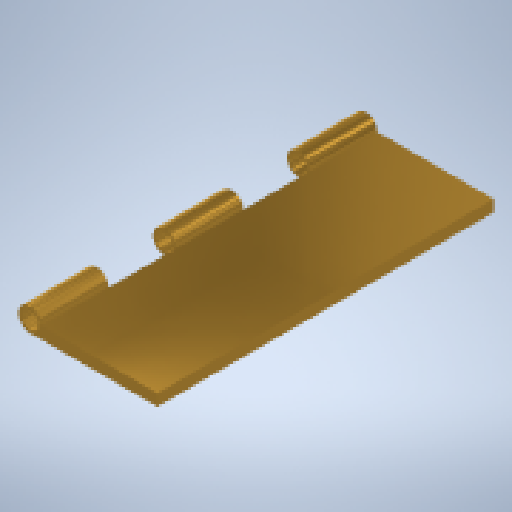
# Autodesk Inventor part: SchnierTeilA
Saved by Autodesk Inventor 2024 (Build 280153000, 153)
## iProperties
Created: 2023-11-30
Part Number: SchnierTeilA
Material: Generic
Document SubType Name: Modeling
Designer: Daniel Nussbaum
Density: 1 g/cm^3
Appearance: Default
Author: Daniel Nussbaum
Autodesk Inventor part; units mm, degrees
ref_plane "YZ Plane" through (0, 0, 0) normal (1, 0, 0) x (0, 1, 0)
ref_plane "XZ Plane" through (0, 0, 0) normal (0, 1, 0) x (-1, 0, 0)
ref_plane "XY Plane" through (0, 0, 0) normal (0, 0, 1) x (1, 0, 0)
sketch "Sketch1" plane through (0, 0, 0) normal (0, 0, 1) x (1, 0, 0)
  line L0 (0, 0) -> (-20, 0)
  line L1 (-20, 0) -> (-20, 2)
  line L2 (-20, 2) -> (0, 2)
  line L3 (0, 2) -> (0, 0)
  line L4 (-20, 2) -> (-22, 2)
  line L5 (-22, 2) -> (-22, 4)
  circle A0 centre (-22, 2) radius 2
  line L6 (-22, 0) -> (-20, 0)
  dimension "d0" = 20
  dimension "d1" = 2
  dimension "d2" = 2
  dimension "d3" = 2
  constraints: 14 end point, 2 horizontal, 2 parallel, 2 perpendicular, 2 point on circle, 1 centre point, 1 coincident, 1 tangent
  measures "d0" distance of L1.end L2.end
  measures "d1" distance of L0.end L1.end
  measures "d2" distance of L1.end L4.end
  measures "d3" distance of L4.end L5.end
extrude "Extrusion1" add sketch "Sketch1" along normal blind 58
sketch "Sketch2" plane through (-20, 2, 0) normal (0, 1, 0) x (1, 0, 0)
  line L0 (0, 0) -> (-2, 0) projected
  line L1 (-2, 0) -> (-2, -58) projected
  line L2 (0, -58) -> (-2, -58) projected
  line L3 (0, 0) -> (0, -58) projected
  line L4 (20, 0) -> (0, 0) projected
  line L5 (0, 0) -> (0, -58) projected
  line L6 (20, -58) -> (0, -58) projected
  line L7 (20, 0) -> (20, -58) projected
  line L8 (-4, -58) -> (0, -58) projected
  line L9 (-4, -58) -> (0, -58)
  line L10 (0, -58) -> (0, -46.4)
  line L11 (0, -46.4) -> (-4, -46.4)
  line L12 (-4, -46.4) -> (-4, -58)
  line L13 (-4, -46.4) -> (0, -46.4)
  line L14 (0, -46.4) -> (0, -34.8)
  line L15 (0, -34.8) -> (-4, -34.8)
  line L16 (-4, -34.8) -> (-4, -46.4)
  line L17 (-4, 0) -> (-4, -58) projected
  line L18 (0, -34.8) -> (-4, -34.8)
  line L19 (-4, -34.8) -> (-4, -23.2)
  line L20 (-4, -23.2) -> (0, -23.2)
  line L21 (0, -23.2) -> (0, -34.8)
  line L22 (-4, -23.2) -> (0, -23.2)
  line L23 (0, -23.2) -> (0, -11.6)
  line L24 (0, -11.6) -> (-4, -11.6)
  line L25 (-4, -11.6) -> (-4, -23.2)
  line L26 (0, -11.6) -> (-4, -11.6)
  line L27 (-4, -11.6) -> (-4, 0)
  line L28 (-4, 0) -> (0, 0)
  line L29 (0, 0) -> (0, -11.6)
  point P0 (0, -11.6)
  point P1 (-4, -11.6)
  point P2 (0, -23.2)
  dimension "d6" = 11.6
  dimension "d7" = 11.6
  dimension "d8" = 11.6
  dimension "d9" = 11.6
  constraints: 40 end point, 10 parallel, 5 horizontal, 5 perpendicular, 5 point on line
  measures "d6" distance of L10.end L9.end
  measures "d7" distance of L14.end L13.end
  measures "d8" distance of L18.end L19.end
  measures "d9" distance of L23.end L22.end
extrude "Extrusion2" cut sketch "Sketch2" along normal mid plane 4 contours L3 L20 L1 L24 | L1 L20 L17 L24 | L3 L11 L1 L15 | L1 L11 L16 L15
sketch "Sketch3" plane through (0, 0, 58) normal (0, 0, 1) x (1, 0, 0)
  line L0 (-22, 0) -> (0, 0) projected
  line L1 (0, 0) -> (0, 2) projected
  line L2 (0, 2) -> (-20, 2) projected
  arc A0 (-20, 2) -> (-22, 0) centre (-22, 2) ccw projected
hole "Hole1" at (-22, 2, 58) direction (0, 0, -1) diameter 3 end through all
body "Solid1"
